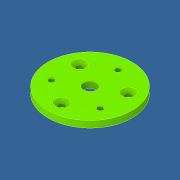
# Autodesk Inventor part: GripperMountCover
Saved by Autodesk Inventor 2016 (Build 200138000, 138)
## iProperties
Created: 2016-03-29
Part Number: GripperMountCover
Material: ABS-Kunststoff
Document SubType Name: Modeling
Designer: 4ndreas
Density: 1.06 g/cm^3
Appearance: Glatt - grün
Mass: 3.51856 g
Surface Area: 28.0326 cm^2
Volume: 3.3194 cm^3
Author: 4ndreas
Autodesk Inventor part; units mm, degrees
ref_plane "YZ Plane" through (0, 0, 0) normal (1, 0, 0) x (0, 1, 0)
ref_plane "XZ Plane" through (0, 0, 0) normal (0, 1, 0) x (-1, 0, 0)
ref_plane "XY Plane" through (0, 0, 0) normal (0, 0, 1) x (1, 0, 0)
sketch "Skizze1" plane through (0, 0, 0) normal (0, 0, 1) x (1, 0, 0)
  circle A0 centre (0, 13) radius 1.25 projected
  circle A1 centre (0, -13) radius 1.25 projected
  circle A2 centre (11.2583, 6.5) radius 1.25 projected
  circle A3 centre (11.2583, -6.5) radius 1.25 projected
  circle A4 centre (-11.2583, 6.5) radius 1.25 projected
  circle A5 centre (-11.2583, -6.5) radius 1.25 projected
  arc A6 (-8.7265, -12.2003) -> (-6.2025, -13.6575) centre (0, 0) ccw projected
  arc A7 (-8.9067, -9.0923) -> (-8.7265, -12.2003) centre (-7.563, -10.5736) ccw projected
  arc A8 (-8.9067, -9.0923) -> (-12.3275, -3.1673) centre (-11.2583, -6.5) ccw projected
  arc A9 (-14.929, -1.4572) -> (-12.3275, -3.1673) centre (-12.9385, -1.2629) ccw projected
  arc A10 (-14.929, 1.4572) -> (-14.929, -1.4572) centre (0, 0) ccw projected
  arc A11 (-12.3275, 3.1673) -> (-14.929, 1.4572) centre (-12.9385, 1.2629) ccw projected
  arc A12 (-12.3275, 3.1673) -> (-8.9067, 9.0923) centre (-11.2583, 6.5) ccw projected
  arc A13 (-8.7265, 12.2003) -> (-8.9067, 9.0923) centre (-7.563, 10.5736) ccw projected
  arc A14 (-6.2025, 13.6575) -> (-8.7265, 12.2003) centre (0, 0) ccw projected
  arc A15 (-3.4208, 12.2596) -> (-6.2025, 13.6575) centre (-5.3755, 11.8365) ccw projected
  arc A16 (-3.4208, 12.2596) -> (3.4208, 12.2596) centre (0, 13) ccw projected
  arc A17 (6.2025, 13.6575) -> (3.4208, 12.2596) centre (5.3755, 11.8365) ccw projected
  arc A18 (8.7265, 12.2003) -> (6.2025, 13.6575) centre (0, 0) ccw projected
  arc A19 (8.9067, 9.0923) -> (8.7265, 12.2003) centre (7.563, 10.5736) ccw projected
  arc A20 (8.9067, 9.0923) -> (12.3275, 3.1673) centre (11.2583, 6.5) ccw projected
  arc A21 (14.929, 1.4572) -> (12.3275, 3.1673) centre (12.9385, 1.2629) ccw projected
  arc A22 (14.929, -1.4572) -> (14.929, 1.4572) centre (0, 0) ccw projected
  arc A23 (12.3275, -3.1673) -> (14.929, -1.4572) centre (12.9385, -1.2629) ccw projected
  arc A24 (12.3275, -3.1673) -> (8.9067, -9.0923) centre (11.2583, -6.5) ccw projected
  arc A25 (8.7265, -12.2003) -> (8.9067, -9.0923) centre (7.563, -10.5736) ccw projected
  arc A26 (6.2025, -13.6575) -> (8.7265, -12.2003) centre (0, 0) ccw projected
  arc A27 (3.4208, -12.2596) -> (6.2025, -13.6575) centre (5.3755, -11.8365) ccw projected
  arc A28 (3.4208, -12.2596) -> (-3.4208, -12.2596) centre (0, -13) ccw projected
  arc A29 (-6.2025, -13.6575) -> (-3.4208, -12.2596) centre (-5.3755, -11.8365) ccw projected
  circle A30 centre (0, 0) radius 17.5 projected
  circle A31 centre (0, 0) radius 19.42 projected
  circle A32 centre (0, 0) radius 3
  point P0 (0, 0)
  dimension "d0" = 6
  constraints: 1 centre point, 1 coincident
  measures "d0" diameter of A32
extrude "Extrusion1" add sketch "Skizze1" along normal blind 3 contours A7 A8 A9 A10 A11 A12 A13 A14 A15 A16 A17 A18 A19 A20 A21 A22 A23 A24 A25 A26 A27 A28 A29 A6 | A30 | A31
sketch "Skizze2" plane through (0, 0, 3) normal (0, 0, 1) x (1, 0, 0)
  circle A0 centre (0, 0) radius 3 projected
  circle A1 centre (-11.2583, -6.5) radius 1.25 projected
  circle A2 centre (-11.2583, 6.5) radius 1.25 projected
  circle A3 centre (11.2583, -6.5) radius 1.25 projected
  circle A4 centre (11.2583, 6.5) radius 1.25 projected
  circle A5 centre (0, -13) radius 1.25 projected
  circle A6 centre (0, 13) radius 1.25 projected
  circle A7 centre (0, 0) radius 19.42 projected
  point P0 (0, 0)
hole "Bohrung1" at (-11.2583, 6.5, 3) at (0, -13, 3) at (11.2583, 6.5, 3) direction (0, 0, -1) diameter 3 end through all countersink diameter 6 countersink angle 90
